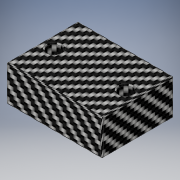
# Autodesk Inventor part: enginefoot
Saved by Autodesk Inventor 2017 (Build 210142000, 142)
## iProperties
Created: 2020-01-04
Part Number: enginefoot
Material: Steel, Carbon
Document SubType Name: Modeling
Designer: Admin
Density: 7.85 g/cm^3
Appearance: Carbon Fiber
Author: Admin
Autodesk Inventor part; units mm, degrees
ref_plane "YZ Plane" through (0, 0, 0) normal (1, 0, 0) x (0, 1, 0)
ref_plane "XZ Plane" through (0, 0, 0) normal (0, 1, 0) x (-1, 0, 0)
ref_plane "XY Plane" through (0, 0, 0) normal (0, 0, 1) x (1, 0, 0)
sketch "Sketch1" plane through (0, 0, 0) normal (0, 1, 0) x (-1, 0, 0)
  line L0 (-12.7, -9.525) -> (12.7, -9.525)
  line L1 (12.7, -9.525) -> (12.7, 9.525)
  line L2 (12.7, 9.525) -> (-12.7, 9.525)
  line L3 (-12.7, 9.525) -> (-12.7, -9.525)
  line L4 (-12.7, -9.525) -> (12.7, 9.525) construction
  line L5 (12.7, -9.525) -> (-12.7, 9.525) construction
  circle A0 centre (9.525, 0) radius 1.7859
  circle A1 centre (-9.525, 0) radius 1.7859
  point P0 (0, 0)
  dimension "d0" = 25.4
  dimension "d1" = 19.05
  dimension "d2" = 3.5719
  dimension "d3" = 3.5719
  dimension "d4" = 19.05
  dimension "d5" = 3.175
  dimension "d6" = 3.175
  dimension "d7" = 5.715
  constraints: 12 end point, 2 centre point, 2 midpoint, 2 parallel, 1 horizontal, 1 perpendicular
  measures "d0" distance of L2.end L1.end
  measures "d1" distance of L0.end L1.end
  measures "d2" diameter of A0
  measures "d3" diameter of A1
  measures "d4" distance of A0.centre A1.centre
  measures "d5" distance from line of L3 A1.centre
  measures "d6" distance from line of A0.centre L1
  measures "d7" distance from line of A0.centre L4
extrude "Extrusion1" add sketch "Sketch1" along normal mid plane 9.525
fillet "Fillet1" radius 0.3175 16 edges at (11.3109, -4.7625, 0) (11.3109, 4.7625, 0) (-7.7391, -4.7625, 0) (-7.7391, 4.7625, 0) (0, -4.7625, -9.525) (12.7, -4.7625, 0) (0, -4.7625, 9.525) (-12.7, -4.7625, 0) (12.7, 0, -9.525) (12.7, 4.7625, 0) (12.7, 0, 9.525) (0, 4.7625, 9.525) (-12.7, 0, 9.525) (-12.7, 4.7625, 0) (-12.7, 0, -9.525) (0, 4.7625, -9.525)
body "Solid1"
